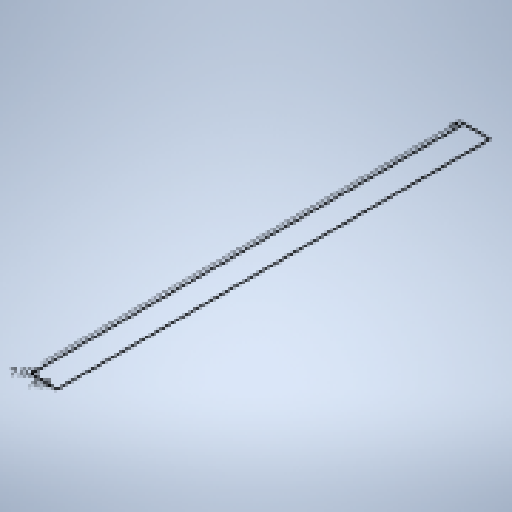
# Autodesk Inventor part: battery shim
Saved by Autodesk Inventor 2023 (Build 270158000, 158)
## iProperties
Created: 2023-02-08
Part Number: battery shim
Material: Generic
Document SubType Name: Modeling
Designer: Gabriel - T3 CAD
Density: 1 g/cm^3
Appearance: Default
Author: Gabriel - T3 CAD
Autodesk Inventor part; units mm, degrees
ref_plane "YZ Plane" through (0, 0, 0) normal (1, 0, 0) x (0, 1, 0)
ref_plane "XZ Plane" through (0, 0, 0) normal (0, 1, 0) x (-1, 0, 0)
ref_plane "XY Plane" through (0, 0, 0) normal (0, 0, 1) x (1, 0, 0)
sketch "Sketch1" plane through (0, 0, 0) normal (0, 1, 0) x (-1, 0, 0)
  line L0 (0, 0) -> (10.922, 0)
  line L1 (10.922, 0) -> (10.922, 181.102)
  line L2 (10.922, 181.102) -> (0, 181.102)
  line L3 (0, 181.102) -> (0, 0)
  dimension "d0" = 10.922
  dimension "d1" = 181.102
  constraints: 8 end point, 2 parallel, 1 horizontal, 1 perpendicular
  measures "d0" distance of L2.end L1.end
  measures "d1" distance of L1.end L0.end
extrude "Extrusion1" add sketch "Sketch1" along normal blind 50.8
sketch "Sketch2" plane through (0, 0, 181.102) normal (1, 0, 0) x (0, 0, -1)
  circle A0 centre (39.751, 25.4) radius 3.9688
  circle A1 centre (141.351, 25.4) radius 3.9688
  line L0 (0, 0) -> (181.102, 0) projected
  line L1 (181.102, 0) -> (181.102, 50.8) projected
  circle A2 centre (39.751, 25.4) radius 2.5797
  circle A3 centre (141.351, 25.4) radius 2.5797
  dimension "d4" = 7.9375
  dimension "d5" = 7.9375
  dimension "d6" = 0
  dimension "d7" = 25.4
  dimension "d8" = 101.6
  dimension "d9" = 39.751
  dimension "d10" = 5.1594
  dimension "d11" = 5.1594
  constraints: 4 centre point, 2 coincident
  measures "d4" diameter of A1
  measures "d5" diameter of A0
  measures "d6" vertical distance of A1.centre A0.centre
  measures "d7" distance from line of L0 A1.centre
  measures "d8" distance of A0.centre A1.centre
  measures "d9" distance from line of L1 A1.centre
  measures "d10" diameter of A2
  measures "d11" diameter of A3
extrude "Extrusion2" cut sketch "Sketch2" against normal blind 50.8 contours A2 | A3
extrude "Extrusion3" cut sketch "Sketch2" against normal blind 5.1594 contours A0 | A1 | A2 | A3
equation "\"d5\" = d4"
body "Solid1"
